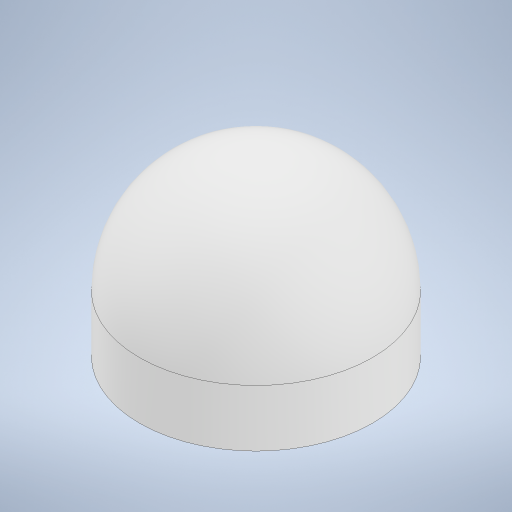
# Autodesk Inventor part: Cap
Saved by Autodesk Inventor 2023 (Build 270158030, 158C)
## iProperties
Created: 2022-09-17
Part Number: Cap
Material: PVC-Piping
Document SubType Name: Modeling
Designer: cjj5381
Density: 1.4 g/cm^3
Appearance: Smooth - White
Author: cjj5381
Autodesk Inventor part; units mm, degrees
ref_plane "YZ Plane" through (0, 0, 0) normal (1, 0, 0) x (0, 1, 0)
ref_plane "XZ Plane" through (0, 0, 0) normal (0, 1, 0) x (-1, 0, 0)
ref_plane "XY Plane" through (0, 0, 0) normal (0, 0, 1) x (1, 0, 0)
sketch "Sketch1" plane through (0, 0, 0) normal (1, 0, 0) x (0, 1, 0)
  arc A0 (0, -78.0796) -> (78.0796, 0) centre (0, 0) ccw
  line L0 (0, -78.0796) -> (-38.1, -78.0796)
  line L1 (-38.1, -78.0796) -> (-38.1, -71.5264)
  line L2 (-38.1, -71.5264) -> (0, -71.5264)
  arc A1 (0, -71.5264) -> (71.5264, 0) centre (0, 0) ccw
  line L3 (0, 0) -> (85.8053, 0)
  line L4 (78.0796, 0) -> (71.5264, 0)
  dimension "d1" = 38.1
  dimension "d2" = 6.5532
  dimension "d4" = 71.5264
  constraints: 10 end point, 4 point on circle, 2 centre point, 2 coincident, 2 horizontal, 2 point on line, 2 tangent, 1 perpendicular, 1 vertical
  measures "d1" distance of L0.start L0.end
  measures "d2" distance of L0.end L1.end
  measures "d4" radius of A1
revolve "Revolution1" add sketch "Sketch1" angle 360 about axis through (0, 0, 0) along (0, 1, 0)
body "Solid1"
